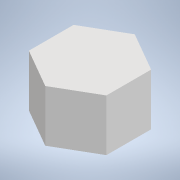
# Autodesk Inventor part: Part3
Saved by Autodesk Inventor 2021 (Build 250183000, 183)
## iProperties
Created: 2022-03-11
Part Number: Part3
Material: Generic
Document SubType Name: Modeling
Designer: Norbert_Prokopiuk
Mass: 997661 g
Surface Area: 58196.9 cm^2
Volume: 997661 cm^3
Density: 1 g/cm^3
Appearance: Default
Author: Norbert_Prokopiuk
Autodesk Inventor part; units mm, degrees
ref_plane "YZ Plane" through (0, 0, 0) normal (1, 0, 0) x (0, 1, 0)
ref_plane "XZ Plane" through (0, 0, 0) normal (0, 1, 0) x (-1, 0, 0)
ref_plane "XY Plane" through (0, 0, 0) normal (0, 0, 1) x (1, 0, 0)
sketch "Sketch1" plane through (0, 0, 0) normal (0, 1, 0) x (-1, 0, 0)
  line L0 (0, -692.8203) -> (-600, -346.4102)
  line L1 (-600, -346.4102) -> (-600, 346.4102)
  line L2 (-600, 346.4102) -> (0, 692.8203)
  line L3 (0, 692.8203) -> (600, 346.4102)
  line L4 (600, 346.4102) -> (600, -346.4102)
  line L5 (600, -346.4102) -> (0, -692.8203)
  point P0 (0, 0)
  point P1 (0, 0)
  dimension "d0" = 1200
  constraints: 12 end point, 1 coincident, 13 other
  measures "d0" distance between parallel lines of L1 L4
extrude "Extrusion1" add sketch "Sketch1" along normal blind 800
sketch "Sketch2" plane through (600, 0, 346.4102) normal (0.5, 0, 0.866) x (0.866, 0, -0.5)
  line L0 (-692.8203, 0) -> (-692.8203, 800) projected
  line L1 (-692.8203, 400) -> (0, 400)
  line L2 (0, 0) -> (0, 800) projected
  point P0 (-346.4102, 0)
  dimension "d3" = 400
  constraints: 2 end point, 2 midpoint, 1 horizontal
  measures "d3" distance from line of point (-346.41, 0) L1
sketch "Sketch3" plane through (600, 0, 346.4102) normal (1, 0, 0) x (0, 0, -1)
  line L0 (0, 0) -> (0, 800) projected
  line L1 (0, 400) -> (692.8203, 400)
  line L2 (692.8203, 0) -> (692.8203, 800) projected
  point P0 (346.4102, 0)
  constraints: 2 end point, 2 midpoint
sketch "Sketch4" plane through (0, 0, -692.8203) normal (0.5, 0, -0.866) x (-0.866, 0, -0.5)
  line L0 (-692.8203, 0) -> (-692.8203, 800) projected
  line L1 (-692.8203, 400) -> (0, 400)
  line L2 (0, 0) -> (0, 800) projected
  point P0 (-346.4102, 0)
  constraints: 2 end point, 2 midpoint
sketch "Sketch5" plane through (0, 0, 692.8203) normal (-0.5, 0, 0.866) x (0.866, 0, 0.5)
  line L0 (0, 400) -> (-692.8203, 400) projected
  point P0 (-346.4102, 0)
sketch "Sketch6" plane through (-600, 0, -346.4102) normal (-1, 0, 0) x (0, 0, 1)
  line L0 (692.8203, 400) -> (0, 400) projected
  point P0 (346.4102, 0)
sketch "Sketch7" plane through (-600, 0, -346.4102) normal (-0.5, 0, -0.866) x (-0.866, 0, 0.5)
  line L0 (0, 400) -> (-692.8203, 400) projected
  point P0 (-346.4102, 0)
body "Solid1"
